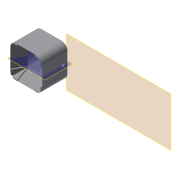
# Autodesk Inventor part: 10_OPENTRONS_LED_FLUO_MODULE
Saved by Autodesk Inventor 2019.4 (Build 234330000, 330)
## iProperties
Created: 2021-02-25
Part Number: 10_OPENTRONS_LED_FLUO_MODULE
Material: Generic
Document SubType Name: Modeling
Designer: diederichbenedict
Density: 1 g/cm^3
Appearance: Default
Author: diederichbenedict
Autodesk Inventor part; units mm, degrees
ref_plane "YZ Plane" through (0, 0, 0) normal (1, 0, 0) x (0, 1, 0)
ref_plane "XZ Plane" through (0, 0, 0) normal (0, 1, 0) x (-1, 0, 0)
ref_plane "XY Plane" through (0, 0, 0) normal (0, 0, 1) x (1, 0, 0)
ref_plane "Work Plane1" through (0, 0, 0) normal (0, 0, 1) x (1, 0, 0)
sketch "Sketch1" plane through (0, 0, 0) normal (0, 0, 1) x (1, 0, 0)
  circle A0 centre (-34.5766, 0) radius 11 projected
  line L0 (-42.9814, 7.8492) -> (-37.1719, 11.2033)
  line L1 (-18, -19) -> (-18, 19) projected
  line L2 (-23.5766, 3.3541) -> (-23.5766, -3.3541)
  line L3 (-37.1719, -11.2033) -> (-42.9814, -7.8492)
  arc A1 (-42.9814, 7.8492) -> (-42.9814, -7.8492) centre (-34.5766, 0) ccw
  arc A2 (-37.1719, -11.2033) -> (-23.5766, -3.3541) centre (-34.5766, 0) ccw
  arc A3 (-23.5766, 3.3541) -> (-37.1719, 11.2033) centre (-34.5766, 0) ccw
  line L4 (-21.0766, 13.5) -> (-48.0766, 13.5)
  line L5 (-48.0766, 13.5) -> (-48.0766, -13.5)
  line L6 (-48.0766, -13.5) -> (-21.0766, -13.5)
  line L7 (-21.0766, -13.5) -> (-21.0766, 13.5)
  line L8 (-21.0766, 13.5) -> (-48.0766, -13.5) construction
  line L9 (-48.0766, 13.5) -> (-21.0766, -13.5) construction
  point P0 (0, 0)
  point P1 (-34.5766, 0)
  dimension "d4" = 27
  dimension "d5" = 27
  constraints: 18 end point, 6 point on circle, 3 centre point, 3 midpoint, 3 parallel, 2 coincident, 1 horizontal, 1 perpendicular, 1 tangent, 1 other
  measures "d4" distance of L6.end L5.end
  measures "d5" distance of L5.end L4.end
extrude "Extrusion1" add sketch "Sketch1" along normal blind 12
sketch "Sketch2" plane through (-48.0766, -13.5, 0) normal (0, -1, 0) x (1, 0, 0)
  line L0 (0, 0) -> (27, 0) projected
  line L1 (27, 0) -> (27, 12) projected
  line L2 (0, 12) -> (27, 12) projected
  line L3 (0, 0) -> (0, 12) projected
  line L4 (0, 12) -> (0, 21.3932)
  line L5 (27, 12) -> (0, 12) projected
  line L6 (0, 12) -> (3.5944, 12)
  line L7 (0, 12) -> (5.135, 12)
  line L8 (2.2643, 17.6594) -> (16.3015, 26.1722)
  line L9 (0, 21.3932) -> (5.135, 12)
  point P0 (48.0766, 0)
  constraints: 10 end point, 2 point on line, 1 vertical
extrude "Extrusion2" add sketch "Sketch2" against normal up to surface (27 mm away) contours L4 L9 L2
sketch "Sketch4" plane through (-48.0766, -13.5, 21.3932) normal (0.8774462, 0, 0.4796751) x (0.4796751, 0, -0.8774462)
  line L0 (2.5, 12) -> (2.5, 17) construction
  line L1 (2.5, 17) -> (7.5, 17) construction
  line L2 (7.5, 17) -> (7.5, 12) construction
  line L3 (7.5, 12) -> (2.5, 12) construction
  line L4 (0, 22.25) -> (0, 6.75) construction
  line L5 (0, 6.75) -> (10, 6.75) construction
  line L6 (10, 6.75) -> (10, 22.25) construction
  line L7 (10, 22.25) -> (0, 22.25) construction
  line L8 (10.7052, 27) -> (0, 27) projected
  line L9 (0, 0) -> (0, 27) projected
  line L10 (10.7052, 0) -> (0, 0) projected
  line L11 (10.7052, 27) -> (10.7052, 21.3722) projected
  line L12 (10.7052, 5.6278) -> (10.7052, 21.3722) construction
  line L13 (10.7052, 5.6278) -> (10.7052, 0) projected
  line L14 (18.7714, 27) -> (0, 27) projected
  line L15 (0, 27) -> (10, 27)
  line L16 (10, 27) -> (10, 21)
  line L17 (10, 21) -> (0, 21)
  line L18 (0, 21) -> (0, 27)
  line L19 (0, 0) -> (0, 27) projected
  line L20 (0, 0) -> (10, 0)
  line L21 (10, 0) -> (10, 6)
  line L22 (10, 6) -> (0, 6)
  line L23 (0, 6) -> (0, 0)
  point P0 (41.8325, 13.5)
  dimension "d19" = 6
  dimension "d20" = 6
  constraints: 16 end point, 4 parallel, 2 horizontal, 2 perpendicular, 1 point on line
  measures "d19" distance of L15.end L16.end
  measures "d20" distance of L21.end L20.end
extrude "Extrusion4" add sketch "Sketch4" along normal blind 1
pattern_circular "Circular Pattern1" count 4 over 360 about axis through (-34.5766, 0, 0) along (0, 0, 1) of "Extrusion2", "Extrusion4"
fillet "Fillet1" radius 5 4 edges at (-48.0766, -13.5, 10.6966) (-21.0766, -13.5, 10.6966) (-21.0766, 13.5, 10.6966) (-48.0766, 13.5, 10.6966)
ref_plane "Work Plane2" through (-43.0766, 0, 0) normal (0, -1, 0) x (1, 0, 0)
sketch "Sketch5" plane through (-48.0766, -7.5, 21.3932) normal (-1, 0, 0) x (0, 0, 1)
  line L0 (4.8543, 7.5) -> (-25.7678, 7.5) projected
  circle A0 centre (-17.9445, 7.5) radius 1.4
  point P0 (-21.3932, 7.5)
  dimension "d21" = 2.8
  constraints: 1 centre point, 1 point on line
  measures "d21" diameter of A0
extrude "Extrusion5" cut sketch "Sketch5" against normal through all
equation "\"d22\" = d21"
body "Solid1"
